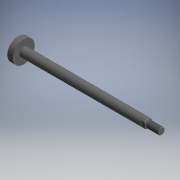
# Autodesk Inventor part: CP96S40-160_ROD
Saved by Autodesk Inventor 2017.3 (Build 213256000, 256)
## iProperties
Part Number: CP96S40-160_ROD
Material: Generic
Catalog Web Link: www.cadenas.de
Description: CP96 ROD-ISO Cylinder:Standard Double Acting,Single/Double Rod
Vendor: SMC
Document SubType Name: Modeling
Designer: partserver
Manufacturer: SMC
Mass: 60.7941 g
Surface Area: 160.851 cm^2
Volume: 60.7941 cm^3
Density: 1 g/cm^3
Appearance: PSOLRGB-128-128-128
Category: PARTsolutions
Company: SMC
Title: CP96S40-160_ROD
Author: Cadenas PARTsolutions
Comments: ISO Cylinder:Standard Double Acting,Single/Double Rod
PSOL_IDENT_0: {$CADENAS_DATA\23d-libs\smc_jp\actuator\standard_air_cylinder\cp96_c96\cp96\parts\cp96_rod.prj},193
PSOL_IDENT_1: {VTYP=3D},{NB=CP96S40-160_ROD},{LINA=CP96S40-160_ROD},{NN=CP96 ROD},{DATE=18.06.2021 10:30:56},{GEOM
PSOL_IDENT_2: DATE=30.10.2018 03:42:00},{VERSION=},{LINEID=20},{WBVAR=STROKE,ROD,BOOT},{WBNUMERIC=STROKE}  {NB=CP9
PSOL_IDENT_3: 6S40-160_ROD},{LINA=CP96S40-160_ROD},{KT=DUMMY},{BORE=40},{STROKE=160},{ROD=},{BOOT=},{BOOTX='','(-)
PSOL_IDENT_4: Without boot','J','(J) Nylon tarpaulin (one end)','K','(K) Heat resistant tarpaulin (one end)'},{OR
PSOL_IDENT_5: DER=CP96S40-160},{A=24},{B=35},{D=16},{L12=6.5},{KK=M12x1.25},{KKRA=12},{KKRP=1.25},{SW=13},{G=37.5}
PSOL_IDENT_6: ,{L8=105},{H=54},{RR=2},{LD1=14},{A1=2.00},{LD2=10.4},{HB=113},{HB1=75.000},{HB2=88.000},{HB3=100.00
PSOL_IDENT_7: 0},{HB4=113.000},{HB5=138.000},{HB6=163.000},{HB7=188.000},{HB8=213.000},{HB9=238.000},{HB10=263.000
PSOL_IDENT_8: },{HB11=288.000},{HB12=313.000}
NB: CP96S40-160_ROD
NN: CP96 ROD
NT: ISO Cylinder:Standard Double Acting,Single/Double Rod
NBSYN: $ORDER._ROD
LINA: CP96S40-160_ROD
CATALOG: SMC (JP
BORE: 40
STROKE: 160
ROD: (-) Single rod
BOOT: (-) Without boot
A: 24
B: 35
D: 16
L12: 6.5
KK: M12x1.25
SW: 13
G: 37.5
L8: 105
H: 54
RR: 2
LD1: 14
HB1: 75
HB2: 88
HB3: 100
HB4: 113
HB5: 138
HB6: 163
HB7: 188
HB8: 213
HB9: 238
HB10: 263
HB11: 288
HB12: 313
SUPPLIER: SMC
ARTICLENO: CP96S40-160_ROD
BOMINFO: CP96S40-160_ROD
CREATOR: CADENAS GmbH
Autodesk Inventor part; units mm, degrees
ref_plane "YZ Plane" through (0, 0, 0) normal (1, 0, 0) x (0, 1, 0)
ref_plane "XZ Plane" through (0, 0, 0) normal (0, 1, 0) x (-1, 0, 0)
ref_plane "XY Plane" through (0, 0, 0) normal (0, 0, 1) x (1, 0, 0)
sketch "Sketch_9" plane through (0, 0, 0) normal (0, 0, 1) x (1, 0, 0)
  line L0 (207.5, 0) -> (-54, 0)
  line L1 (-54, 0) -> (-54, 5.233)
  line L2 (-54, 5.233) -> (-53.233, 6)
  line L3 (-53.233, 6) -> (-32.767, 6)
  line L4 (-32.767, 6) -> (-32, 5.233)
  line L5 (-32, 5.233) -> (-32, 5.2)
  line L6 (-32, 5.2) -> (-30, 5.2)
  line L7 (-30, 5.2) -> (-30, 7)
  line L8 (-30, 7) -> (-28.2679, 8)
  line L9 (-28.2679, 8) -> (197.5, 8)
  line L10 (197.5, 8) -> (197.5, 20)
  line L11 (197.5, 20) -> (207.5, 20)
  line L12 (207.5, 20) -> (207.5, 0)
  line L13 (207.5, 0) -> (-54, 0)
  constraints: 28 end point
revolve "Revolution1" add sketch "Sketch_9" angle 360 about axis through (207.5, 0, 0) along (1, 0, 0)
thread "Thread1" size "M12x1.25" class "6g" standard "ISO Metric profile" full length
sketch "Sketch_4" plane through (-30, 0, 0) normal (1, 0, 0) x (0, 0, -1)
  line L0 (-15, -11.5) -> (15, -11.5)
  line L1 (15, -11.5) -> (15, 11.5)
  line L2 (15, 11.5) -> (-15, 11.5)
  line L3 (-15, 11.5) -> (-15, -11.5)
  line L4 (-10, 6.5) -> (-10, -6.5)
  line L5 (-10, -6.5) -> (10, -6.5)
  line L6 (10, -6.5) -> (10, 6.5)
  line L7 (10, 6.5) -> (-10, 6.5)
  constraints: 16 end point
extrude "Extrusion1" cut sketch "Sketch_4" along normal blind 6.5
ref_plane "A4_XY" through (455, 0, 0) normal (0, 1, 0) x (1, 0, 0)
ref_plane "A4_YZ" through (455, 0, 0) normal (1, 0, 0) x (0, 0, -1)
ref_plane "A4_ZX" through (455, 0, 0) normal (0, 0, -1) x (0, 1, 0)
ref_plane "ROD_BODY_XY" through (0, 0, 0) normal (1, 0, 0) x (0, 0, -1)
ref_plane "ROD_BODY_YZ" through (0, 0, 0) normal (0, 0, -1) x (0, 1, 0)
ref_plane "ROD_BODY_ZX" through (0, 0, 0) normal (0, 1, 0) x (1, 0, 0)
ref_plane "ROD_NUT_XY" through (-54, 0, 0) normal (-1, 0, 0) x (0, 0, -1)
ref_plane "ROD_NUT_YZ" through (-54, 0, 0) normal (0, 0, -1) x (0, -1, 0)
ref_plane "ROD_NUT_ZX" through (-54, 0, 0) normal (0, -1, 0) x (-1, 0, 0)
body "Solid1"
